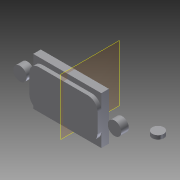
# Autodesk Inventor part: DB9 connector 2017_06_14
Saved by Autodesk Inventor 2012 (Build 160160000, 160)
## iProperties
Created: 2017-04-26
Part Number: DB9 connector 2017_06_14
Material: Default
Document SubType Name: Modeling
Designer: Brandon
Density: 1 g/cm^3
Author: Brandon
Autodesk Inventor part; units mm, degrees
ref_plane "XZ Plane" through (0, 0, 0) normal (0, 1, 0) x (-1, 0, 0)
ref_plane "XY Plane" through (0, 0, 0) normal (0, 0, 1) x (1, 0, 0)
sketch "Sketch1" plane through (0, 0, 0) normal (0, 0, 1) x (1, 0, 0)
  line L0 (-9, 12.55) -> (9, 12.55)
  line L1 (9, 12.55) -> (9, 0)
  line L2 (9, 0) -> (-9, 0)
  line L3 (-9, 0) -> (-9, 12.55)
  circle A0 centre (-12.495, 6.275) radius 1.7859
  circle A1 centre (12.495, 6.275) radius 1.7859
  point P0 (0, 0)
  dimension "d0" = 18
  dimension "d1" = 12.55
  dimension "d2" = 9
  dimension "d3" = 0
  dimension "d14" = 24.99
  dimension "d15" = 12.495
  dimension "d16" = 6.275
  dimension "d17" = 6.275
  dimension "d18" = 3.5719
  dimension "d19" = 3.5719
  constraints: 8 end point, 2 centre point, 2 parallel, 1 horizontal, 1 perpendicular
  measures "d0" distance of L1.end L2.end
  measures "d1" distance of L0.end L1.end
  measures "d2" distance from line of point (0, 0) L1
  measures "d3" distance from line of L2 point (0, 0)
  measures "d14" distance of A1.centre A0.centre
  measures "d15" horizontal distance of point (0, 0) A0.centre
  measures "d16" distance from line of A0.centre L2
  measures "d17" distance from line of L2 A1.centre
  measures "d18" diameter of A0
  measures "d19" diameter of A1
extrude "Extrusion1" add sketch "Sketch1" along normal blind 2
sketch "Sketch2" plane through (-9, 0, 0) normal (0, -1, 0) x (1, 0, 0)
  line L0 (18, 0) -> (0, 0) projected
  circle A0 centre (-3.495, -9.5) radius 1.525
  circle A1 centre (21.495, -9.5) radius 1.525
  point P0 (9, 0)
  dimension "d6" = 3.05
  dimension "d7" = 3.05
  dimension "d8" = 24.99
  dimension "d9" = 12.495
  dimension "d10" = 9.5
  dimension "d11" = 9.5
  constraints: 2 centre point
  measures "d6" diameter of A0
  measures "d7" diameter of A1
  measures "d8" distance of A1.centre A0.centre
  measures "d9" horizontal distance of point (9, 0) A1.centre
  measures "d10" distance from line of L0 A0.centre
  measures "d11" distance from line of L0 A1.centre
extrude "Extrusion2" add sketch "Sketch2" along normal blind 1
sketch "Sketch3" plane through (0, 0, 2) normal (0, 0, 1) x (1, 0, 0)
  line L0 (9, 12.55) -> (9, 0) projected
  line L1 (-9, 0) -> (-9, 12.55) projected
  line L2 (9, 0) -> (-9, 0) projected
  line L3 (-6.5, 11.275) -> (6.5, 11.275)
  line L4 (9, 8.775) -> (9, 3.775)
  line L5 (6.5, 1.275) -> (-6.5, 1.275)
  line L6 (-9, 3.775) -> (-9, 8.775)
  arc A0 (-6.5, 11.275) -> (-9, 8.775) centre (-6.5, 8.775) ccw
  arc A1 (9, 8.775) -> (6.5, 11.275) centre (6.5, 8.775) ccw
  arc A2 (6.5, 1.275) -> (9, 3.775) centre (6.5, 3.775) ccw
  arc A3 (-9, 3.775) -> (-6.5, 1.275) centre (-6.5, 3.775) ccw
  point P0 (0, 0)
  point P1 (-9, 11.275)
  point P2 (9, 1.275)
  point P3 (9, 11.275)
  dimension "d20" = 10
  dimension "d21" = 1.275
  dimension "d22" = 12.55
  dimension "d23" = 2.5
  constraints: 8 end point, 8 point on circle, 8 point on line, 8 tangent, 4 centre point, 3 equal radius, 2 parallel, 1 horizontal, 1 perpendicular
  measures "d20" distance of point (9, 11.275) point (9, 1.275)
  measures "d21" distance between parallel lines of L5 L2
  measures "d22" distance of L1.start L1.end
  measures "d23" radius of A0
extrude "Extrusion3" add sketch "Sketch3" along normal blind 1 contours L0 A2 L5 A3 L1 A0 L3 A1
equation "\"d2\" = 0.5 * d0"
equation "\"d15\" = 0.5 * d14"
equation "\"d16\" = 0.5 * d1"
equation "\"d17\" = d16"
equation "\"d9\" = 0.5 * d8"
equation "\"d21\" = -0.5 * d20 + 0.5 * d22"
body "Solid1"
